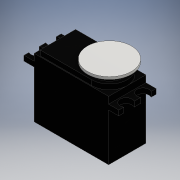
# Autodesk Inventor part: servo
Saved by Autodesk Inventor 2016 (Build 200138000, 138)
## iProperties
Created: 2015-10-07
Part Number: servo
Material: Generic
Document SubType Name: Modeling
Designer: alex
Density: 1 g/cm^3
Appearance: Default
Mass: 38.0536 g
Surface Area: 85.0823 cm^2
Volume: 38.0536 cm^3
Author: alex
Autodesk Inventor part; units mm, degrees
ref_plane "YZ Plane" through (0, 0, 0) normal (1, 0, 0) x (0, 1, 0)
ref_plane "XZ Plane" through (0, 0, 0) normal (0, 1, 0) x (-1, 0, 0)
ref_plane "XY Plane" through (0, 0, 0) normal (0, 0, 1) x (1, 0, 0)
sketch "Sketch1" plane through (0, 0, 0) normal (0, 1, 0) x (-1, 0, 0)
  line L0 (-22, 17.5) -> (22, 17.5)
  line L1 (22, 17.5) -> (22, -17.5)
  line L2 (22, -17.5) -> (-22, -17.5)
  line L3 (-22, -17.5) -> (-22, 17.5)
  line L4 (-22, 17.5) -> (22, -17.5) construction
  line L5 (22, 17.5) -> (-22, -17.5) construction
  point P0 (0, 0)
  dimension "d0" = 44
  dimension "d1" = 35
  constraints: 12 end point, 2 midpoint, 2 parallel, 1 horizontal, 1 perpendicular
  measures "d0" distance of L1.end L2.end
  measures "d1" distance between parallel lines of L2 L0
extrude "Extrusion1" add sketch "Sketch1" along normal mid plane 22
sketch "Sketch2" plane through (-22, 11, 17.5) normal (0, 0, 1) x (1, 0, 0)
  line L0 (3, -0.5) -> (44, -0.5)
  line L1 (44, -0.5) -> (44, -21.5)
  line L2 (44, -21.5) -> (3, -21.5)
  line L3 (3, -21.5) -> (3, -0.5)
  line L4 (0, 0) -> (0, -22) projected
  line L5 (44, 0) -> (0, 0) projected
  line L6 (0, -22) -> (44, -22) projected
  line L7 (44, 0) -> (44, -22) projected
  point P0 (22, -11)
  dimension "d4" = 3
  dimension "d5" = 0.5
  dimension "d6" = 0.5
  dimension "d7" = 0
  constraints: 8 end point, 2 parallel, 1 horizontal, 1 perpendicular
  measures "d4" distance between parallel lines of L4 L3
  measures "d5" distance between parallel lines of L5 L0
  measures "d6" distance between parallel lines of L6 L2
  measures "d7" distance between parallel lines of L7 L1
extrude "Extrusion2" add sketch "Sketch2" along normal blind 3 contours L0 L1 L2 L3
fillet "Fillet1" radius 10.5 1 edges at (22, 10.5, 19)
fillet "Fillet2" radius 10.5 1 edges at (22, -10.5, 19)
sketch "Sketch3" plane through (-22, 11, 20.5) normal (0, 0, 1) x (1, 0, 0)
  circle A0 centre (33.5, -11) radius 8.5
  arc A1 (33.5, -21.5) -> (33.5, -0.5) centre (33.5, -11) ccw projected
  point P0 (22, -11)
  dimension "d13" = 2
  constraints: 1 centre point, 1 concentric
  measures "d13" radial gap between concentric circles of A1 A0
extrude "Extrusion3" add sketch "Sketch3" along normal blind 1
sketch "Sketch4" plane through (11.5, 0, 21.5) normal (0, 0, 1) x (1, 0, 0)
  circle A0 centre (0, 0) radius 5.5
  circle A1 centre (0, 0) radius 8.5 projected
  point P0 (-11.5, 0)
  dimension "d16" = 3
  constraints: 1 centre point, 1 concentric
  measures "d16" radial gap between concentric circles of A1 A0
extrude "Extrusion4" add sketch "Sketch4" along normal blind 3 contours A0
sketch "Sketch5" plane through (11.5, 0, 24.5) normal (0, 0, 1) x (1, 0, 0)
  circle A0 centre (0, 0) radius 13
  point P0 (-11.5, 0)
  dimension "d19" = 26
  constraints: 1 centre point
  measures "d19" diameter of A0
extrude "Extrusion5" add sketch "Sketch5" along normal blind 1.5
sketch "Sketch7" plane through (-22, -11, 17.5) normal (-1, 0, 0) x (0, 0, 1)
  line L0 (-4, 22) -> (-7, 22)
  line L1 (-7, 22) -> (-7, 0)
  line L2 (-7, 0) -> (-4, 0)
  line L3 (-4, 0) -> (-4, 22)
  line L4 (0, 22) -> (0, 0) projected
  line L5 (-35, 22) -> (0, 22) projected
  line L6 (-35, 0) -> (0, 0) projected
  point P0 (-17.5, 11)
  dimension "d22" = 4
  dimension "d23" = 3
  dimension "d24" = 0
  dimension "d25" = 0
  constraints: 8 end point, 2 parallel, 1 horizontal, 1 perpendicular
  measures "d22" distance between parallel lines of L3 L4
  measures "d23" distance between parallel lines of L1 L3
  measures "d24" distance between parallel lines of L5 L0
  measures "d25" distance between parallel lines of L6 L2
extrude "Extrusion6" add sketch "Sketch7" along normal blind 6 contours L3 L2 L1 L0
sketch "Sketch8" plane through (-22, -11, 13.5) normal (0, 0, 1) x (1, 0, 0)
  circle A0 centre (-4.3, 16) radius 3.5
  circle A1 centre (-4.3, 6) radius 3.5
  line L0 (0, 0) -> (-6, 0) projected
  line L1 (0, 22) -> (-6, 22) projected
  line L2 (-6, 0) -> (-6, 22) projected
  point P0 (22, 11)
  dimension "d28" = 7
  dimension "d29" = 6
  dimension "d30" = 7
  dimension "d31" = 6
  dimension "d32" = 1.7
  dimension "d33" = 1.7
  constraints: 2 centre point
  measures "d28" diameter of A0
  measures "d29" distance from line of L0 A1.centre
  measures "d30" diameter of A1
  measures "d31" distance from line of L1 A0.centre
  measures "d32" distance from line of L2 A0.centre
  measures "d33" distance from line of L2 A1.centre
extrude "Extrusion7" cut sketch "Sketch8" against normal through all
mirror "Mirror1" about plane through (0, 0, 0) normal (1, 0, 0) of "Extrusion6", "Extrusion7"
body "Solid1"
